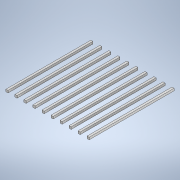
# Autodesk Inventor part: structure1
Saved by Autodesk Inventor 2022 (Build 260153000, 153)
## iProperties
Created: 2022-04-07
Part Number: structure1
Material: Generic
Document SubType Name: Modeling
Designer: ten26
Density: 1 g/cm^3
Appearance: Default
Author: ten26
Autodesk Inventor part; units mm, degrees
ref_plane "YZ Plane" through (0, 0, 0) normal (1, 0, 0) x (0, 1, 0)
ref_plane "XZ Plane" through (0, 0, 0) normal (0, 1, 0) x (-1, 0, 0)
ref_plane "XY Plane" through (0, 0, 0) normal (0, 0, 1) x (1, 0, 0)
sketch "Sketch1" plane through (0, 0, 0) normal (0, 1, 0) x (-1, 0, 0)
  line L0 (1, -40) -> (-1, -40)
  line L1 (-1, -40) -> (-1, 40)
  line L2 (-1, 40) -> (1, 40)
  line L3 (1, 40) -> (1, -40)
  line L4 (1, -40) -> (-1, 40) construction
  line L5 (-1, -40) -> (1, 40) construction
  point P0 (0, 0)
  dimension "d0" = 80
  dimension "d1" = 2
  constraints: 12 end point, 2 midpoint, 2 parallel, 1 horizontal, 1 perpendicular
  measures "d0" distance of L0.end L1.end
  measures "d1" distance of L1.end L2.end
extrude "Extrusion1" add sketch "Sketch1" along normal blind 2.1
pattern_linear "Rectangular Pattern1" count 10 spacing 8.5 along (1, 0, 0) of "Extrusion1"
equation "\"base_add\" = 0.6"
body "Solid1"
